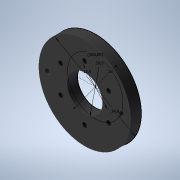
# Autodesk Inventor part: Encoder_Montage
Saved by Autodesk Inventor 2022 (Build 260153000, 153)
## iProperties
Created: 2023-07-28
Part Number: Encoder_Montage
Material: Generisch
Document SubType Name: Modeling
Designer: aewalder
Density: 1 g/cm^3
Appearance: Vorgabe
Author: aewalder
Autodesk Inventor part; units mm, degrees
ref_plane "YZ Plane" through (0, 0, 0) normal (1, 0, 0) x (0, 1, 0)
ref_plane "XZ Plane" through (0, 0, 0) normal (0, 1, 0) x (-1, 0, 0)
ref_plane "XY Plane" through (0, 0, 0) normal (0, 0, 1) x (1, 0, 0)
sketch "Sketch1" plane through (0, 0, 0) normal (0, 0, 1) x (1, 0, 0)
  circle A0 centre (0, 0) radius 17.3
  circle A1 centre (0, 0) radius 14 construction
  line L0 (-14, 0) -> (14, 0) construction
  circle A2 centre (0, 0) radius 10.45 construction
  line L1 (0, 10.45) -> (0, 0) construction
  circle A3 centre (0, 0) radius 6.75
  point P0 (-9.05, 5.225)
  point P1 (-9.05, -5.225)
  point P2 (0, -10.45)
  point P3 (9.05, -5.225)
  point P4 (9.05, 5.225)
  dimension "d2" = 20.9
  dimension "d0" = 34.6
  dimension "d1" = 28
  dimension "d5" = 360
  dimension "d7" = 13.5
  constraints: 4 coincident, 4 end point, 3 centre point, 2 point on circle, 1 horizontal, 1 midpoint, 1 vertical, 1 vertical alignment, 9 other
  measures "d0" diameter of A0
  measures "d1" diameter of A1
  measures "d7" diameter of A3
extrude "Extrusion1" add sketch "Sketch1" along normal blind 4
hole "Hole1" at (14, 0, 0) at (-14, 0, 0) direction (0, 0, 1) diameter 2.2 end through all counterbore diameter 4.4 counterbore depth 0.9 clearance for "Senkschraube mit Linsenkopf ISO 2010" size "M2" standard "DIN"
hole "Hole2" at (0, 10.45, 0) at (-9.05, 5.225, 0) at (-9.05, -5.225, 0) at (0, -10.45, 0) at (9.05, -5.225, 0) at (9.05, 5.225, 0) direction (0, 0, 1) diameter 1.567 end through all thread size "M2x0.4" class "6H" standard "ISO Metric profile"
thicken "Thicken1" operation add thickness 0.15 both sides no extend neighbours yes toward (0.0804666, 0.9967573, 0) faces at (-8.9869, 6.006, 1.3333) (-8.9869, -4.444, 1.3333) (0.063, 11.231, 1.3333) (9.113, 6.006, 1.3333) (9.113, -4.444, 1.3333) (0.063, -9.669, 1.3333)
body "Solid1"
